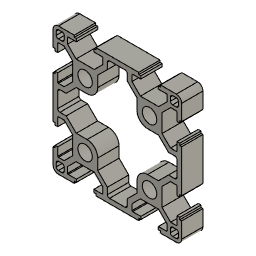
60 x60 Profile v1 (Autodesk Fusion 360 design; units mm, degrees)
Autodesk Fusion 360 part; units mm, degrees
sketch "Sketch1" plane through (0, 0, 0) normal (0, 1, 0) x (1, 0, 0)
  line L0 (29.9708, 29.9124) -> (-30.0292, -29.9708) construction
  line L1 (-28.2363, 28.2363) -> (29.9708, -29.9708) construction
  line L2 (-27.8292, -0.0693) -> (-30.0292, -0.0693)
  line L3 (0.128, 27.8292) -> (0.128, 30.0292)
  line L4 (-10.8831, 27.8292) -> (-10.8831, 29.1292)
  line L5 (-19.0831, 27.8292) -> (-19.0831, 29.1292)
  line L6 (-20.0831, 29.1292) -> (-20.0831, 30.0292)
  line L7 (-9.8831, 29.1292) -> (-9.8831, 30.0292)
  circle A0 centre (-14.9831, 14.9831) radius 3.4
  line L8 (-29.1292, 19.0831) -> (-27.8292, 19.0831)
  line L9 (-29.1292, 10.8831) -> (-27.8292, 10.8831)
  line L10 (-30.0292, 9.8831) -> (-29.1292, 9.8831)
  line L11 (-30.0292, 20.0831) -> (-29.1292, 20.0831)
  line L12 (0.128, 30.0292) -> (-9.8831, 30.0292)
  line L13 (-20.0831, 30.0292) -> (-27.5292, 30.0292)
  line L14 (-20.0831, 29.1292) -> (-19.0831, 29.1292)
  line L15 (-10.8831, 29.1292) -> (-9.8831, 29.1292)
  line L16 (-19.0831, 27.8292) -> (-22.932, 27.8292)
  line L17 (-27.8292, 19.0831) -> (-27.8292, 22.9003)
  line L18 (-29.1292, 9.8831) -> (-29.1292, 10.8831)
  line L19 (-29.1292, 19.0831) -> (-29.1292, 20.0831)
  line L20 (-30.0292, 27.5292) -> (-30.0292, 20.0831)
  line L21 (-30.0292, 9.8831) -> (-30.0292, -0.0693)
  line L22 (-9.072, 19.293) -> (-4.5331, 23.8231)
  line L23 (-24.7708, 6.7331) -> (-20.8292, 10.667)
  line L24 (-23.8607, 4.5331) -> (-19.1611, 9.2236)
  line L25 (-9.072, 14.2236) -> (-9.072, 19.293)
  line L26 (-20.8292, 10.667) -> (-20.8292, 19.1979)
  line L27 (-19.2305, 20.7862) -> (-10.6927, 20.7837)
  line L28 (-30.0292, -0.0693) -> (0.128, 30.0292) construction
  line L29 (-19.1611, 9.2236) -> (-14.072, 9.2236)
  line L30 (-23.2331, 24.7887) -> (-19.2305, 20.7862)
  line L31 (-24.8501, 23.2023) -> (-20.8292, 19.1979)
  line L32 (-26.8292, 4.5331) -> (-23.8607, 4.5331)
  line L33 (-27.5292, 6.7331) -> (-24.7708, 6.7331)
  line L34 (-27.5295, 23.2003) -> (-24.8501, 23.2023)
  line L35 (-27.8292, 7.0331) -> (-27.8292, 10.8831)
  line L36 (-4.5331, 23.8231) -> (-4.5331, 26.8292)
  line L37 (-6.7331, 24.7356) -> (-6.7331, 27.5292)
  line L38 (-10.6927, 20.7837) -> (-6.7331, 24.7356)
  line L39 (-23.2331, 24.7887) -> (-23.232, 27.5293)
  arc A1 (-14.072, 9.2236) -> (-9.072, 14.2236) centre (-14.072, 14.2236) ccw
  line L40 (0.128, 27.8292) -> (-3.5331, 27.8292)
  line L41 (-7.0331, 27.8292) -> (-10.8831, 27.8292)
  line L42 (-27.8292, 2.1265) -> (-27.8292, 3.5331)
  arc A2 (-26.8292, 4.5331) -> (-27.8292, 3.5331) centre (-26.8292, 3.5331) ccw
  arc A3 (-3.5331, 27.8292) -> (-4.5331, 26.8292) centre (-3.5331, 26.8292) ccw
  arc A4 (-6.7331, 27.5292) -> (-7.0331, 27.8292) centre (-7.0331, 27.5292) ccw
  arc A5 (-22.932, 27.8292) -> (-23.232, 27.5293) centre (-22.932, 27.5292) ccw
  arc A6 (-27.5295, 23.2003) -> (-27.8292, 22.9003) centre (-27.5292, 22.9003) ccw
  arc A7 (-27.8292, 7.0331) -> (-27.5292, 6.7331) centre (-27.5292, 7.0331) ccw
  line L43 (-27.5292, 28.5292) -> (-25.7792, 28.5292)
  line L44 (-24.7792, 27.5292) -> (-24.7792, 25.7792)
  line L45 (-25.7792, 24.7792) -> (-27.5292, 24.7792)
  line L46 (-28.5292, 25.7792) -> (-28.5292, 27.5292)
  arc A8 (-25.7792, 24.7792) -> (-24.7792, 25.7792) centre (-25.7792, 25.7792) ccw
  arc A9 (-28.5292, 25.7792) -> (-27.5292, 24.7792) centre (-27.5292, 25.7792) ccw
  arc A10 (-27.5292, 28.5292) -> (-28.5292, 27.5292) centre (-27.5292, 27.5292) ccw
  arc A11 (-24.7792, 27.5292) -> (-25.7792, 28.5292) centre (-25.7792, 27.5292) ccw
  arc A12 (-27.5292, 30.0292) -> (-30.0292, 27.5292) centre (-27.5292, 27.5292) ccw
  line L47 (-27.8292, -0.0693) -> (-27.8292, 2.1265)
  point P0 (-30.0292, 30.0292)
  point P1 (-28.5292, 28.5292)
  point P2 (-24.7792, 24.7792)
  point P3 (-28.5292, 24.7792)
  dimension "d1" = 60
  dimension "d2" = 60.0001
  dimension "d3" = 60
  dimension "d4" = 60
  dimension "d5" = 2.2
  dimension "d7" = 6.8
  dimension "d8" = 21.1893
  dimension "d9" = 4.1
  dimension "d10" = 4.1
  dimension "d11" = 1
  dimension "d12" = 1
  dimension "d13" = 4.1
  dimension "d14" = 4.1
  dimension "d15" = 1
  dimension "d16" = 1
  dimension "d17" = 0.9
  dimension "d18" = 0.9
  dimension "d19" = 9.2
  dimension "d20" = 9.2
  dimension "d23" = 1.1
  dimension "d24" = 1.1
  dimension "d25" = 1.1
  dimension "d26" = 1.1
  dimension "d29" = 8.25
  dimension "d32" = 8.25
  dimension "d33" = 2.2
  dimension "d34" = 2.2
  dimension "d35" = 5
  dimension "d36" = 1
  dimension "d37" = 0.3
  dimension "d38" = 3.75
  dimension "d39" = 3.75
  dimension "d40" = 1.5
  dimension "d41" = 1.5
  dimension "d42" = 1
  dimension "d43" = 2.5
  constraint horizontal L12
  constraint perpendicular L12 L20
  constraint coincident L0 origin
  constraint coincident L1 origin
  constraint perpendicular L2 L20
  constraint perpendicular L3 L12
  constraint perpendicular L20 L40
  constraint perpendicular L4 L12
  constraint perpendicular L5 L12
  constraint coincident L6.end L12
  constraint perpendicular L6 L12
  constraint perpendicular L7 L12
  constraint coincident L1 A0.centre
  constraint perpendicular L11 L18
  constraint perpendicular L7 L14
  constraint collinear L12 L13
  constraint collinear L14 L15
  constraint collinear L16 L40
  constraint coincident L10.start L20
  constraint collinear L18 L19
  constraint collinear L20 L21
  constraint parallel L23 L24
  constraint parallel L0 L22
  constraint parallel L0 L38
  constraint parallel L0 L24
  constraint perpendicular L25 L29
  constraint perpendicular L12 L37
  constraint perpendicular L12 L36
  constraint tangent L25 A1
  constraint tangent L29 A1
  constraint collinear L40 L41
  constraint coincident L28 L42.start
  constraint tangent L32 A2
  constraint tangent L42 A2
  constraint tangent L36 A3
  constraint tangent L40 A3
  constraint equal A2 A3
  constraint tangent L37 A4
  constraint tangent L41 A4
  constraint tangent L39 A5
  constraint tangent L16 A5
  constraint equal A4 A5
  constraint tangent L34 A6
  constraint tangent L17 A6
  constraint equal A4 A6
  constraint tangent L33 A7
  constraint tangent L35 A7
  constraint equal A4 A7
  constraint horizontal L43
  constraint vertical L44
  constraint horizontal L45
  constraint vertical L46
  constraint coincident L1 P1
  constraint coincident P2 L44
  constraint coincident P2 L45
  constraint tangent L44 A8
  constraint tangent L45 A8
  constraint coincident P3 L45
  constraint coincident P3 L46
  constraint tangent L45 A9
  constraint tangent L46 A9
  constraint equal A8 A9
  constraint coincident P1 L43
  constraint coincident P1 L46
  constraint tangent L43 A10
  constraint tangent L46 A10
  constraint equal A8 A10
  constraint tangent L43 A11
  constraint tangent L44 A11
  constraint equal A8 A11
  constraint coincident A10 L1.start
  constraint coincident P0 L13
  constraint coincident P0 L20
  constraint tangent L13 A12
  constraint tangent L20 A12
  constraint perpendicular L2 L47
  measures "d1" distance of L0.end L1.end
  measures "d2" distance of L0.start P0
  measures "d3" distance of P0 L0.end
  measures "d4" distance of P0 L0.end
  measures "d5" distance of L12 L40
  measures "d7" diameter of A0
  measures "d8" distance of origin A0.centre
  measures "d9" distance of L4 A0.centre
  measures "d10" distance of L5 A0.centre
  measures "d11" distance of L5 L6
  measures "d12" distance of L4 L7
  measures "d13" distance of A0.centre L9
  measures "d14" distance of A0.centre L8
  measures "d15" distance of L8 L11
  measures "d16" distance of L9 L10
  measures "d17" distance of L12 L14
  measures "d18" distance of L18 L20
  measures "d19" distance of L21 L26
  measures "d20" distance of L3 L25
  measures "d23" distance of L23 L28
  measures "d24" distance of L24 L28
  measures "d25" distance of L28 L38
  measures "d26" distance of L22 L28
  measures "d29" distance of A0.centre L33
  measures "d32" distance of A0.centre L37
  measures "d33" distance of L36 L37
  measures "d34" distance of L32 L33
  measures "d35" radius of A1
  measures "d36" radius of A2
  measures "d37" radius of A4
  measures "d38" distance of P2 P3
  measures "d39" distance of P1 P3
  measures "d40" distance of L20 L46
  measures "d41" distance of L13 L43
  measures "d42" radius of A8
  measures "d43" radius of A12
extrude "Extrude1" add sketch "Sketch1" along normal blind 10 makes body 1
mirror "Mirror1" about plane through (0.128, 0, -27.8292) normal (-1, 0, 0) of bodies 1 merged
mirror "Mirror2" about plane through (-27.8292, 0, 0.0693) normal (0, 0, 1) of bodies 1 merged
copy_body "Body->Comp1" bodies 1 removing the originals makes body 2 in component "60 x 60 Profile"
component "60 x 60 Profile" placed x (1, 0, 0) y (0, 1, 0) z (0, 0, 1) at (0, 0, 0)
